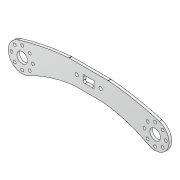
# Autodesk Inventor part: 16_012_FEMUR_FRAME_DRIVER_R1
Saved by Autodesk Inventor 2021.2 (Build 252289000, 289)
## iProperties
Created: 2020-07-26
Part Number: 16_012_FEMUR_FRAME_DRIVER_R1
Material: Aluminum 6061
Document SubType Name: Modeling
Designer: y6tada
Density: 2.7 g/cm^3
Appearance: Aluminum - Flat
Author: y6tada
Autodesk Inventor part; units mm, degrees
ref_plane "YZ Plane" through (0, 0, 0) normal (1, 0, 0) x (0, 1, 0)
ref_plane "XZ Plane" through (0, 0, 0) normal (0, 1, 0) x (-1, 0, 0)
ref_plane "XY Plane" through (0, 0, 0) normal (0, 0, 1) x (1, 0, 0)
sketch "Sketch1" plane through (0, 0, 0) normal (0, 0, 1) x (1, 0, 0)
  line L0 (0, 0) -> (100, 0) construction
  arc A0 (10.5, 0) -> (-3.0807, 10.0379) centre (0, 0) ccw construction
  arc A1 (89.5, 0) -> (95.0588, -9.2647) centre (100, 0) ccw construction
  arc A2 (95.0588, -9.2647) -> (60.7485, 1.3948) centre (50, -93.75) ccw
  arc A3 (103.0807, 10.0379) -> (64.7857, 17.3948) centre (50, -162.9167) ccw
  line L1 (35.2143, 17.3948) -> (64.7857, 17.3948)
  line L2 (39.2515, 1.3948) -> (60.7485, 1.3948)
  line L3 (50, 0) -> (50, 2) construction
  line L4 (50, 18) -> (50, 2) construction
  line L5 (35.2143, 17.3948) -> (39.2515, 1.3948) construction
  line L6 (0, 0) -> (37.2329, 9.3948) construction
  arc A4 (39.2515, 1.3948) -> (4.9412, -9.2647) centre (50, -93.75) ccw
  arc A5 (60.7485, 1.3948) -> (39.2515, 1.3948) centre (50, -93.75) ccw construction
  arc A6 (35.2143, 17.3948) -> (-3.0807, 10.0379) centre (50, -162.9167) ccw
  arc A7 (64.7857, 17.3948) -> (35.2143, 17.3948) centre (50, -162.9167) ccw construction
  arc A8 (4.9412, -9.2647) -> (10.5, 0) centre (0, 0) ccw construction
  arc A9 (-3.0807, 10.0379) -> (4.9412, -9.2647) centre (0, 0) ccw
  arc A10 (103.0807, 10.0379) -> (89.5, 0) centre (100, 0) ccw construction
  arc A11 (95.0588, -9.2647) -> (103.0807, 10.0379) centre (100, 0) ccw
  dimension "d0" = 100
  dimension "d1" = 21
  dimension "d2" = 2
  dimension "d3" = 16
  dimension "d30" = 16
  dimension "d31" = 38.3998
  constraints: 28 point on circle, 14 end point, 12 centre point, 4 tangent, 3 horizontal, 2 coincident, 2 midpoint, 2 perpendicular, 2 point on line, 1 collinear, 1 equal radius
  measures "d0" distance of L0.start L0.end
  measures "d1" diameter of A0
  measures "d2" distance of L3.start L3.end
  measures "d3" distance of L4.start L3.end
  measures "d30" distance between parallel lines of L1 L2
  measures "d31" distance of L6.start L6.end
extrude "Extrusion1" add sketch "Sketch1" along normal blind 2
sketch "Sketch2" plane through (0, 0, 2) normal (0, 0, 1) x (1, 0, 0)
  line L0 (64.7857, 17.3948) -> (35.2143, 17.3948) construction
  line L1 (39.2515, 1.3948) -> (60.7485, 1.3948) construction
  line L2 (50, 17.3948) -> (50, 1.3948) construction
  line L3 (41, 9.3948) -> (59, 9.3948) construction
  line L4 (46, 6.8448) -> (54, 6.8448)
  line L5 (54, 6.8448) -> (54, 11.9448)
  line L6 (54, 11.9448) -> (46, 11.9448)
  line L7 (46, 11.9448) -> (46, 6.8448)
  line L8 (46, 6.8448) -> (54, 11.9448) construction
  line L9 (54, 6.8448) -> (46, 11.9448) construction
  point P0 (0, 0)
  point P1 (50, 9.3948)
  dimension "d7" = 18
  dimension "d8" = 5.1
  dimension "d9" = 8
  constraints: 16 end point, 6 midpoint, 2 coincident, 2 horizontal, 2 parallel, 1 perpendicular
  measures "d7" distance of L3.start L3.end
  measures "d8" distance of L4.end L5.end
  measures "d9" distance of L5.end L6.end
extrude "Extrusion2" cut sketch "Sketch2" against normal through all
hole "Hole1" at (41, 9.3948, 2) at (59, 9.3948, 2) direction (0, 0, -1) diameter 2.6 end through all
sketch "Sketch3" plane through (0, 0, 2) normal (0, 0, 1) x (1, 0, 0)
  line L0 (46, 11.9448) -> (54, 11.9448) construction
  line L1 (46, 6.8448) -> (46, 11.9448) construction
  line L2 (54, 6.8448) -> (46, 6.8448) construction
  line L3 (54, 11.9448) -> (54, 6.8448) construction
  line L4 (53.2929, 11.2377) -> (46.7071, 11.2377) construction
  line L5 (46.7071, 11.2377) -> (46.7071, 7.5519) construction
  line L6 (46.7071, 7.5519) -> (53.2929, 7.5519) construction
  line L7 (53.2929, 7.5519) -> (53.2929, 11.2377) construction
  circle A0 centre (46.7071, 11.2377) radius 1
  circle A1 centre (46.7071, 7.5519) radius 1
  circle A2 centre (53.2929, 7.5519) radius 1
  circle A3 centre (53.2929, 11.2377) radius 1
  point P0 (0, 0)
  dimension "d19" = 2
  constraints: 8 end point, 4 coincident, 15 other
extrude "Extrusion3" cut sketch "Sketch3" against normal through all
sketch "Sketch4" plane through (0, 0, 2) normal (0, 0, 1) x (1, 0, 0)
  arc A0 (95.0588, -9.2647) -> (103.0807, 10.0379) centre (100, 0) ccw construction
  point P0 (0, 0)
  point P1 (0, 0)
  constraints: 2 coincident
hole "Hole2" at (0, 0, 2) at (100, 0, 2) direction (0, 0, -1) diameter 8 end through all
sketch "Sketch5" plane through (0, 0, 2) normal (0, 0, 1) x (1, 0, 0)
  circle A0 centre (0, 0) radius 8 construction
  circle A1 centre (100, 0) radius 4 construction
  circle A2 centre (100, 0) radius 8 construction
  line L0 (-8, 0) -> (0, 0) construction
  line L1 (100, 0) -> (108, 0) construction
  point P0 (-5.6569, -5.6569)
  point P1 (0, -8)
  point P2 (5.6569, -5.6569)
  point P3 (8, 0)
  point P4 (5.6569, 5.6569)
  point P5 (0, 8)
  point P6 (-5.6569, 5.6569)
  point P7 (105.6569, 5.6569)
  point P8 (100, 8)
  point P9 (94.3431, 5.6569)
  point P10 (92, 0)
  point P11 (94.3431, -5.6569)
  point P12 (100, -8)
  point P13 (105.6569, -5.6569)
  dimension "d36" = 16
  dimension "d34" = 360
  dimension "d39" = 360
  constraints: 4 end point, 3 coincident, 2 horizontal, 2 horizontal alignment, 22 other
hole "Hole3" at (-8, 0, 2) at (-5.6569, -5.6569, 2) at (0, -8, 2) at (5.6569, -5.6569, 2) at (8, 0, 2) at (5.6569, 5.6569, 2) at (0, 8, 2) at (-5.6569, 5.6569, 2) at (108, 0, 2) at (105.6569, 5.6569, 2) at (100, 8, 2) at (94.3431, 5.6569, 2) at (92, 0, 2) at (94.3431, -5.6569, 2) at (100, -8, 2) at (105.6569, -5.6569, 2) direction (0, 0, -1) diameter 2.2 end through all
fillet "Fillet1" radius 3 4 edges at (35.2143, 17.3948, 1) (64.7857, 17.3948, 1) (60.7485, 1.3948, 1) (39.2515, 1.3948, 1)
sketch "Sketch6" plane through (0, 0, 2) normal (0, 0, 1) x (1, 0, 0)
  arc A0 (64.9097, 17.3846) -> (64.6624, 17.3948) centre (64.6624, 14.3948) ccw projected
  line L0 (64.6624, 17.3948) -> (35.3376, 17.3948) projected
  arc A1 (35.3376, 17.3948) -> (35.0903, 17.3846) centre (35.3376, 14.3948) ccw projected
  arc A2 (35.0903, 17.3846) -> (-3.0807, 10.0379) centre (50, -162.9167) ccw projected
  arc A3 (-3.0807, 10.0379) -> (4.9412, -9.2647) centre (0, 0) ccw projected
  arc A4 (39.0796, 1.3752) -> (4.9412, -9.2647) centre (50, -93.75) ccw projected
  arc A5 (39.4217, 1.3948) -> (39.0796, 1.3752) centre (39.4217, -1.6052) ccw projected
  line L1 (39.4217, 1.3948) -> (60.5783, 1.3948) projected
  arc A6 (60.9204, 1.3752) -> (60.5783, 1.3948) centre (60.5783, -1.6052) ccw projected
  arc A7 (95.0588, -9.2647) -> (60.9204, 1.3752) centre (50, -93.75) ccw projected
  arc A8 (95.0588, -9.2647) -> (103.0807, 10.0379) centre (100, 0) ccw projected
  arc A9 (103.0807, 10.0379) -> (64.9097, 17.3846) centre (50, -162.9167) ccw projected
  circle A10 centre (100, -8) radius 1.1 projected
  circle A11 centre (92, 0) radius 1.1 projected
  circle A12 centre (100, 8) radius 1.1 projected
  circle A13 centre (108, 0) radius 1.1 projected
  circle A14 centre (0, 8) radius 1.1 projected
  circle A15 centre (8, 0) radius 1.1 projected
  circle A16 centre (0, -8) radius 1.1 projected
  circle A17 centre (-8, 0) radius 1.1 projected
  circle A18 centre (-5.6569, -5.6569) radius 1.1 projected
  circle A19 centre (5.6569, -5.6569) radius 1.1 projected
  circle A20 centre (5.6569, 5.6569) radius 1.1 projected
  circle A21 centre (-5.6569, 5.6569) radius 1.1 projected
  circle A22 centre (105.6569, 5.6569) radius 1.1 projected
  circle A23 centre (94.3431, 5.6569) radius 1.1 projected
  circle A24 centre (94.3431, -5.6569) radius 1.1 projected
  circle A25 centre (105.6569, -5.6569) radius 1.1 projected
  circle A26 centre (0, 0) radius 4 projected
  circle A27 centre (100, 0) radius 4 projected
  arc A28 (52.5858, 6.8448) -> (54, 8.259) centre (53.2929, 7.5519) ccw projected
  line L2 (52.5858, 6.8448) -> (47.4142, 6.8448) projected
  arc A29 (46, 8.259) -> (47.4142, 6.8448) centre (46.7071, 7.5519) ccw projected
  line L3 (46, 8.259) -> (46, 10.5306) projected
  arc A30 (47.4142, 11.9448) -> (46, 10.5306) centre (46.7071, 11.2377) ccw projected
  line L4 (47.4142, 11.9448) -> (52.5858, 11.9448) projected
  arc A31 (54, 10.5306) -> (52.5858, 11.9448) centre (53.2929, 11.2377) ccw projected
  line L5 (54, 10.5306) -> (54, 8.259) projected
  circle A32 centre (41, 9.3948) radius 1.3 projected
  circle A33 centre (59, 9.3948) radius 1.3 projected
body "Solid1"
